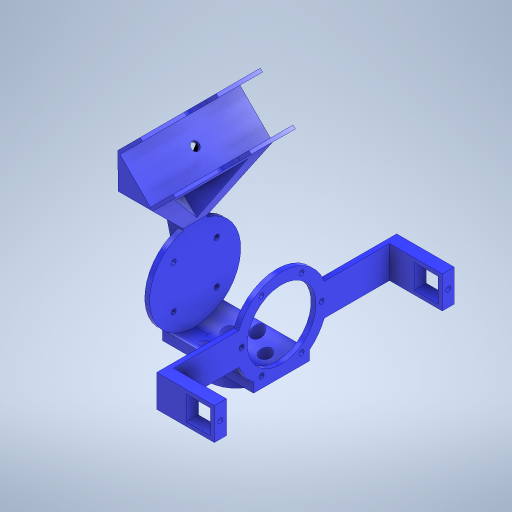
# Autodesk Inventor part: endeff_3dp1
Saved by Autodesk Inventor 2024 (Build 280153000, 153)
## iProperties
Created: 2024-12-14
Part Number: endeff_3dp1
Material: ABS プラスチック
Document SubType Name: Modeling
Designer: hirek
Density: 1.06 g/cm^3
Appearance: 青 - 壁塗料 - 光沢
Author: hirek
Autodesk Inventor part; units mm, degrees
ref_plane "YZ Plane" through (0, 0, 0) normal (1, 0, 0) x (0, 1, 0)
ref_plane "XZ Plane" through (0, 0, 0) normal (0, 1, 0) x (-1, 0, 0)
ref_plane "XY Plane" through (0, 0, 0) normal (0, 0, 1) x (1, 0, 0)
sketch "スケッチ1" plane through (0, 0, 0) normal (1, 0, 0) x (0, 1, 0)
  circle A0 centre (0, 0) radius 28.5
  dimension "d0" = 57
  constraints: 1 centre point, 1 coincident
  measures "d0" diameter of A0
extrude "押し出し1" add sketch "スケッチ1" along normal blind 57
sketch "スケッチ2" plane through (57, 0, 0) normal (1, 0, 0) x (0, 0, -1)
  line L0 (-17.5, 0) -> (17.5, 0)
  line L1 (17.5, 0) -> (17.5, -28.5)
  line L2 (17.5, -28.5) -> (-17.5, -28.5)
  line L3 (-17.5, -28.5) -> (-17.5, 0)
  point P0 (0, 0)
  dimension "d3" = 35
  dimension "d4" = 28.5
  dimension "d5" = 17.5
  dimension "d8" = 0
  constraints: 8 end point, 2 parallel, 1 horizontal, 1 perpendicular
  measures "d3" distance of L1.end L2.end
  measures "d4" distance of L0.end L1.end
  measures "d5" distance from line of point (0, 0) L3
  measures "d8" distance from line of L0 point (0, 0)
extrude "押し出し2" add sketch "スケッチ2" against normal blind 57
sketch "スケッチ3" plane through (57, -28.5, -17.5) normal (0, -1, 0) x (1, 0, 0)
  line L0 (-57, 17.5) -> (0, 17.5)
  line L1 (0, -11) -> (0, 46) projected
  circle A0 centre (-28.5, 17.5) radius 17.5
  point P0 (0, 0)
  point P1 (0, 35)
  dimension "d9" = 35
  constraints: 2 end point, 2 midpoint, 1 centre point
  measures "d9" diameter of A0
extrude "押し出し3" add sketch "スケッチ3" along normal blind 8
sketch "スケッチ4" plane through (57, 0, 0) normal (1, 0, 0) x (0, 0, -1)
  circle A0 centre (0, 0) radius 28.5
  constraints: 1 centre point, 1 coincident
extrude "押し出し4" cut sketch "スケッチ4" against normal blind 54
sketch "スケッチ5" plane through (57, 0, 0) normal (1, 0, 0) x (0, 0, -1)
  circle A0 centre (0, 0) radius 28.5
  constraints: 1 centre point, 1 coincident
extrude "押し出し5" add sketch "スケッチ5" against normal blind 3
sketch "スケッチ6" plane through (28.5, -36.5, 0) normal (0, -1, 0) x (1, 0, 0)
  circle A0 centre (0, 0) radius 13.5
  point P0 (-28.5, 0)
  point P1 (0, -13.5)
  point P2 (11.6913, -6.75)
  point P3 (11.6913, 6.75)
  point P4 (0, 13.5)
  point P5 (-11.6913, 6.75)
  point P6 (-11.6913, -6.75)
  dimension "d16" = 27
  dimension "d19" = 360
  constraints: 1 vertical alignment, 9 other
hole "穴1" at (28.5, -36.5, -13.5) at (40.1913, -36.5, -6.75) at (40.1913, -36.5, 6.75) at (28.5, -36.5, 13.5) at (16.8087, -36.5, 6.75) at (16.8087, -36.5, -6.75) direction (0, 1, 0) diameter 3.2 end through all
sketch "スケッチ7" plane through (0, -28.5, -17.5) normal (0, -1, 0) x (1, 0, 0)
  circle A0 centre (16.8087, 10.75) radius 1.6 projected
  circle A1 centre (28.5, 4) radius 1.6 projected
  circle A2 centre (40.1913, 10.75) radius 1.6 projected
  circle A3 centre (40.1913, 24.25) radius 1.6 projected
  circle A4 centre (28.5, 31) radius 1.6 projected
  circle A5 centre (16.8087, 24.25) radius 1.6 projected
  point P0 (0, 17.5)
  constraints: 6 coincident
hole "穴2" at (16.8087, -28.5, 6.75) at (16.8087, -28.5, -6.75) at (28.5, -28.5, -13.5) at (40.1913, -28.5, -6.75) at (40.1913, -28.5, 6.75) at (28.5, -28.5, 13.5) direction (0, 1, 0) diameter 7.5 end through all
sketch "スケッチ8" plane through (16.8087, -28.5, -6.75) normal (0, 1, 0) x (1, 0, 0)
  circle A0 centre (0, -13.5) radius 1.6 projected
  circle A1 centre (11.6913, -20.25) radius 1.6 projected
  circle A2 centre (23.3827, -13.5) radius 1.6 projected
  circle A3 centre (23.3827, 0) radius 1.6 projected
  circle A4 centre (11.6913, 6.75) radius 1.6 projected
  point P0 (-16.8087, -6.75)
  point P1 (0, 0)
  constraints: 5 coincident
hole "穴3" at (16.8087, -28.5, -6.75) at (16.8087, -28.5, 6.75) at (28.5, -28.5, 13.5) at (40.1913, -28.5, 6.75) at (40.1913, -28.5, -6.75) at (28.5, -28.5, -13.5) direction (0, -1, 0) diameter 7.5 depth 5
sketch "スケッチ9" plane through (0, 0, 0) normal (-1, 0, 0) x (0, 0, 1)
  line L0 (0, 0) -> (20.1525, -20.1525)
  arc A0 (17.5, -22.4944) -> (-17.5, -22.4944) centre (0, 0) ccw projected
  line L1 (0, 0) -> (28.5, 0) construction
  circle A1 centre (0, 0) radius 19
  point P0 (13.435, -13.435)
  point P1 (13.435, 13.435)
  point P2 (-13.435, 13.435)
  point P3 (-13.435, -13.435)
  dimension "d43" = 38
  dimension "d42" = 45
  dimension "d46" = 360
  constraints: 4 end point, 1 coincident, 1 equal length, 1 horizontal, 1 point on circle, 1 point on line, 8 other
  measures "d42" angle of L0 L1
hole "穴4" at (0, -13.435, 13.435) at (0, 13.435, 13.435) at (0, 13.435, -13.435) at (0, -13.435, -13.435) direction (1, 0, 0) diameter 3.2 depth 5
sketch "スケッチ10" plane through (57, 0, 0) normal (1, 0, 0) x (0, 0, -1)
  circle A0 centre (0, 0) radius 25
  line L0 (0, 0) -> (12.5, -21.6506)
  line L1 (0, 0) -> (25, 0) construction
  point P0 (12.5, 21.6506)
  point P1 (-12.5, 21.6506)
  point P2 (-25, 0)
  point P3 (-12.5, -21.6506)
  dimension "d55" = 50
  dimension "d56" = 60
  dimension "d59" = 360
  constraints: 4 end point, 2 coincident, 1 equal length, 1 horizontal, 10 other
  measures "d56" angle of L0 L1
hole "穴5" at (57, -21.6506, -12.5) at (57, -21.6506, 12.5) at (57, 0, 25) at (57, 21.6506, 12.5) at (57, 21.6506, -12.5) at (57, 0, -25) direction (-1, 0, 0) diameter 3.2 depth 5
sketch "スケッチ11" plane through (57, 0, 0) normal (1, 0, 0) x (0, 0, -1)
  circle A0 centre (0, 0) radius 21.5
  dimension "d68" = 43
  constraints: 1 centre point, 1 coincident
  measures "d68" diameter of A0
extrude "押し出し6" cut sketch "スケッチ11" against normal blind 8
sketch "スケッチ14" plane through (54, 0, 0) normal (-1, 0, 0) x (0, 0, 1)
  line L0 (75, 10) -> (-75, 10)
  line L1 (-75, 10) -> (-75, -10)
  line L2 (-75, -10) -> (75, -10)
  line L3 (75, -10) -> (75, 10)
  circle A0 centre (0, 0) radius 28.5
  point P0 (-26.688, -10)
  point P1 (-26.688, 10)
  point P2 (26.688, 10)
  point P3 (26.688, -10)
  dimension "d71" = 150
  dimension "d72" = 20
  dimension "d73" = 75
  dimension "d74" = 10
  constraints: 8 end point, 2 parallel, 1 centre point, 1 coincident, 1 horizontal, 1 perpendicular
  measures "d71" distance of L2.end L1.end
  measures "d72" distance of L1.end L0.end
  measures "d73" distance from line of point (0, 0) L3
  measures "d74" distance from line of point (0, 0) L0
extrude "押し出し7" add sketch "スケッチ14" against normal blind 3 contours L3 L2 A0 L0 | A0 L2 L1 L0
sketch "スケッチ15" plane through (57, 0, 0) normal (1, 0, 0) x (0, 0, -1)
  line L0 (-26.688, 10) -> (-75, 10) projected
  line L1 (-75, -10) -> (-26.688, -10) projected
  line L2 (-75, 10) -> (-67.5, 10)
  line L3 (-67.5, 10) -> (-67.5, -10)
  line L4 (-67.5, -10) -> (-75, -10)
  line L5 (-75, -10) -> (-75, 10)
  line L6 (75, -10) -> (75, 10) projected
  line L7 (75, -10) -> (67.5, -10)
  line L8 (67.5, -10) -> (67.5, 10)
  line L9 (67.5, 10) -> (75, 10)
  line L10 (75, 10) -> (75, -10)
  point P0 (0, 0)
  dimension "d77" = 7.5
  dimension "d78" = 7.5
  constraints: 16 end point, 4 parallel, 2 horizontal, 2 perpendicular, 2 point on line
  measures "d77" distance of L3.end L4.end
  measures "d78" distance of L8.end L9.end
extrude "押し出し8" add sketch "スケッチ15" along normal blind 33
sketch "スケッチ16" plane through (54, -10, 75) normal (0, 0, 1) x (1, 0, 0)
  line L0 (18.5, 17.5) -> (33.5, 17.5)
  line L1 (33.5, 17.5) -> (33.5, 2.5)
  line L2 (33.5, 2.5) -> (18.5, 2.5)
  line L3 (18.5, 2.5) -> (18.5, 17.5)
  line L4 (0, 20) -> (36, 20) projected
  line L5 (36, 20) -> (36, 0) projected
  point P0 (-54, 10)
  point P1 (26, 17.5)
  dimension "d81" = 15
  dimension "d82" = 15
  dimension "d83" = 2.5
  dimension "d84" = 2.5
  constraints: 8 end point, 2 parallel, 1 horizontal, 1 midpoint, 1 perpendicular
  measures "d81" distance of L1.end L2.end
  measures "d82" distance of L0.end L1.end
  measures "d83" distance from line of point (26, 17.5) L4
  measures "d84" distance between parallel lines of L5 L1
extrude "押し出し9" cut sketch "スケッチ16" against normal through all
sketch "スケッチ17" plane through (90, 0, 0) normal (1, 0, 0) x (0, 0, -1)
  line L0 (-67.5, 10) -> (-67.5, -10) projected
  line L1 (-67.5, 10) -> (-75, -10)
  line L2 (26.688, 10) -> (75, 10) projected
  line L3 (26.688, -10) -> (67.5, -10) projected
  line L4 (75, 10) -> (67.5, -10)
  point P0 (0, 0)
  point P1 (-71.25, 0)
  point P2 (71.25, 0)
  constraints: 4 end point, 2 midpoint
hole "穴6" at (90, 0, 71.25) at (90, 0, -71.25) direction (-1, 0, 0) diameter 3.2 depth 8 tip angle 118
sketch "スケッチ19" plane through (3, 0, 0) normal (1, 0, 0) x (0, 0, -1)
  line L0 (7.5, 0) -> (-7.5, 0)
  line L1 (-7.5, 0) -> (-7.5, 28.5)
  line L2 (-7.5, 28.5) -> (7.5, 28.5)
  line L3 (7.5, 28.5) -> (7.5, 0)
  point P0 (0, 0)
  dimension "d94" = 15
  dimension "d95" = 28.5
  dimension "d96" = 28.5
  dimension "d99" = 7.5
  constraints: 8 end point, 2 parallel, 1 horizontal, 1 perpendicular
  measures "d94" distance of L1.end L2.end
  measures "d95" distance of L0.end L1.end
  measures "d96" distance from line of point (0, 0) L2
  measures "d99" distance from line of point (0, 0) L1
extrude "押し出し10" add sketch "スケッチ19" against normal blind 10
sketch "スケッチ20" plane through (3, 27.4955, 7.5) normal (0, 0, 1) x (1, 0, 0)
  line L0 (-10, 1.0045) -> (-3, -27.4955)
  line L1 (-3, -27.4955) -> (-10, -27.4955) projected
  line L2 (-3, -27.4955) -> (-10, -27.4955)
  line L3 (-10, -27.4955) -> (-10, 1.0045)
  constraints: 6 end point, 1 collinear, 1 perpendicular
extrude "押し出し11" cut sketch "スケッチ20" against normal through all
sketch "スケッチ21" plane through (3, 27.4955, 7.5) normal (0, 0, 1) x (1, 0, 0)
  line L0 (11, 31.0045) -> (-10.9203, 52.9249)
  line L1 (-10.9203, 52.9249) -> (3.2218, 67.067)
  line L2 (3.2218, 67.067) -> (25.1421, 45.1467)
  line L3 (25.1421, 45.1467) -> (11, 31.0045)
  line L4 (0, 1.0045) -> (-10, 1.0045) projected
  line L5 (51, 1.0045) -> (51, -17.4955) projected
  line L6 (-3, -27.4955) -> (-10, 1.0045) projected
  line L7 (-10.9203, 52.9249) -> (-10, 1.0045)
  line L8 (-10, 1.0045) -> (0, 1.0045)
  line L9 (11, 31.0045) -> (0, 1.0045)
  dimension "d103" = 31
  dimension "d104" = 20
  dimension "d105" = 30
  dimension "d106" = 40
  constraints: 14 end point, 3 equal length, 1 perpendicular
  measures "d103" distance of L1.end L2.end
  measures "d104" distance of L0.end L1.end
  measures "d105" distance from line of L4 L0.start
  measures "d106" distance from line of L5 L0.start
extrude "押し出し12" add sketch "スケッチ21" against normal blind 45
sketch "スケッチ23" plane through (0, 27.4955, 7.5) normal (0, 0, 1) x (1, 0, 0)
  line L0 (3, 1.0045) -> (-7, 1.0045) projected
  line L1 (-7, 1.0045) -> (3, 1.0045)
  line L2 (28.1421, 45.1467) -> (14, 31.0045) projected
  line L3 (3, 1.0045) -> (14, 31.0045)
  line L4 (14, 31.0045) -> (28.1421, 45.1467)
  line L5 (-7.9203, 52.9249) -> (6.2218, 67.067) projected
  line L6 (28.1421, 45.1467) -> (6.2218, 67.067)
  line L7 (-7, 1.0045) -> (-7.9203, 52.9249) projected
  line L8 (6.2218, 67.067) -> (-7.9203, 52.9249)
  line L9 (-7.9203, 52.9249) -> (-7, 1.0045)
  point P0 (0, -27.4955)
  constraints: 12 end point, 3 collinear, 2 perpendicular
extrude "押し出し13" add sketch "スケッチ23" along normal blind 30
sketch "スケッチ25" plane through (3, 0, 0) normal (1, 0, 0) x (0, 0, -1)
  line L0 (37.5, 58.5) -> (-37.5, 58.5) projected
  line L1 (37.5, 28.5) -> (37.5, 80.4203) projected
  line L2 (-37.5, 58.5) -> (37.5, 58.5)
  line L3 (37.5, 58.5) -> (37.5, 28.5)
  line L4 (37.5, 28.5) -> (-37.5, 28.5)
  line L5 (-37.5, 28.5) -> (-37.5, 58.5)
  line L6 (-7.5, 28.5) -> (-7.5, 27.4955) projected
  line L7 (-7.5, 28.5) -> (-37.5, 58.5)
  line L8 (7.5, 27.4955) -> (7.5, 28.5) projected
  line L9 (7.5, 28.5) -> (37.5, 58.5)
  point P0 (0, 0)
  constraints: 12 end point, 2 parallel, 2 perpendicular, 1 horizontal
extrude "押し出し14" cut sketch "スケッチ25" along normal mid plane 43 contours L1 L4 L9 | L7 L4 L5
sketch "スケッチ26" plane through (0, 27.4955, 37.5) normal (0, 0, 1) x (1, 0, 0)
  line L0 (12.5858, 32.4188) -> (-6.5061, 51.5106)
  line L1 (-6.5061, 51.5106) -> (7.636, 65.6528)
  line L2 (7.636, 65.6528) -> (26.7279, 46.5609)
  line L3 (26.7279, 46.5609) -> (12.5858, 32.4188)
  line L4 (14, 31.0045) -> (28.1421, 45.1467) projected
  line L5 (28.1421, 45.1467) -> (6.2218, 67.067) projected
  point P0 (0, -27.4955)
  dimension "d113" = 27
  dimension "d114" = 20
  dimension "d115" = 2
  dimension "d116" = 0
  constraints: 8 end point, 2 parallel, 1 perpendicular
  measures "d113" distance of L1.end L2.end
  measures "d114" distance of L0.end L1.end
  measures "d115" distance between parallel lines of L4 L3
  measures "d116" distance between parallel lines of L5 L2
extrude "押し出し15" cut sketch "スケッチ26" against normal through all
sketch "スケッチ27" plane through (6.2218, 94.5624, -37.5) normal (-0.7071068, 0.7071068, 0) x (-0.7071068, -0.7071068, 0)
  line L0 (0, 0) -> (20, 0) projected
  line L1 (10, 0) -> (10, 75)
  line L2 (0, 75) -> (20, 75) projected
  circle A0 centre (10, 37.5) radius 10
  line L3 (0, 0) -> (0, 75) projected
  line L4 (10, 27.5) -> (0, 27.5)
  line L5 (0, 27.5) -> (0, 47.5)
  line L6 (0, 47.5) -> (10, 47.5)
  line L7 (10, 47.5) -> (10, 27.5)
  line L8 (20, 0) -> (35.2253, 0) projected
  line L9 (22, 0) -> (22, 75)
  line L10 (35.2253, 75) -> (20, 75) projected
  line L11 (20, 0) -> (20, 75) projected
  line L12 (22, 37.5) -> (56.0624, 37.5)
  line L13 (56.0624, 45) -> (56.0624, 30) projected
  ellipse E0 centre (30.9602, 37.5) end of major axis (30.9602, 16) minor radius 15.2028 projected
  line L14 (22, 15) -> (46.163, 37.5)
  line L15 (46.163, 37.5) -> (22, 60)
  point P0 (71.2652, 37.5)
  point P1 (10, 47.5)
  dimension "d119" = 2
  dimension "d120" = 15
  dimension "d121" = 15
  constraints: 18 end point, 7 point on line, 5 midpoint, 2 parallel, 1 horizontal, 1 horizontal alignment, 1 perpendicular, 1 vertical, 4 other
  measures "d119" distance between parallel lines of L9 L11
  measures "d120" distance from line of L14.start L8
  measures "d121" distance from line of L15.end L10
extrude "押し出し16" cut sketch "スケッチ27" against normal blind 45 contours L3 A0 L4 | A0 L1 | L1 A0 E0 | L3 L6 A0 | E0 A0 | L9 E0 L14 | L9 L12 L14 E0 | L9 E0 L15 L12 | L9 L15 E0
sketch "スケッチ28" plane through (12.5858, 59.9142, -37.5) normal (0.7071068, 0.7071068, 0) x (-0.7071068, 0.7071068, 0)
  line L0 (0, 75) -> (27, 75) projected
  line L1 (13.5, 75) -> (13.5, 0)
  line L2 (27, 0) -> (0, 0) projected
  point P0 (-33.4663, 37.5)
  point P1 (13.5, 37.5)
  constraints: 3 midpoint, 2 end point
hole "穴7" at (3.0398, 69.4602, 0) direction (-0.7071068, -0.7071068, 0) diameter 5.2 depth 8 tip angle 118
